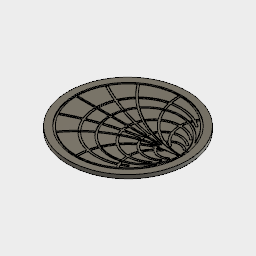
SMITH_FINAL_MODEL v0 (Autodesk Fusion 360 design; units mm, degrees)
Autodesk Fusion 360 part; units mm, degrees
note: some values were not read from the file. Chosen so that the rebuilt part matches the saved one: which face or edge a step refers to; a direction; that a step has no effect; add or cut. Set by a fixed rule: which sketch regions a step uses.
cylinder "CylinderPrimitive1" add diameter 355.6 height 12.7 placed x (1, 0, 0) y (0, 0, -1) z (0, 1, 0) at (0, 0, 0)
sketch "Smith Chart Overlay" plane through (0, 12.7, 0) normal (0, 1, 0) x (-1, 0, 0)
  circle A0 centre (0, 0) radius 177.8
  circle A1 centre (0, 0) radius 177.8
  line L0 (0, 0) -> (-177.8, 0)
  line L1 (0, 0) -> (-118.5333, 0) construction
  line L2 (0, 0) -> (-88.9, 0)
  line L3 (0, 0) -> (-59.2667, 0)
  circle A2 centre (-118.5333, 0) radius 59.2667 construction
  circle A3 centre (-88.9, 0) radius 88.9 construction
  circle A4 centre (-59.2667, 0) radius 118.5333 construction
  arc A5 (-106.68, -142.24) -> (-177.8, 0) centre (-177.8, -88.9) ccw construction
  line L4 (-177.8, 0) -> (-177.8, -88.9)
  line L5 (-177.8, 0) -> (-177.8, 88.9)
  line L6 (-177.8, 177.8) -> (-177.8, 0)
  line L7 (-177.8, 0) -> (-177.8, -177.8)
  line L8 (-177.8, 0) -> (-177.8, -355.6)
  arc A6 (-177.8, 0) -> (-106.68, 142.24) centre (-177.8, 88.9) ccw construction
  arc A7 (0, -177.8) -> (-177.8, 0) centre (-177.8, -177.8) ccw construction
  arc A8 (-177.8, 0) -> (0, 177.8) centre (-177.8, 177.8) ccw construction
  line L9 (-177.8, 355.6) -> (-177.8, 0)
  arc A9 (106.68, -142.24) -> (-177.8, 0) centre (-177.8, -355.6) ccw
  arc A10 (-177.8, 0) -> (106.68, 142.24) centre (-177.8, 355.6) ccw construction
  line L10 (-13.7583, 0) -> (-73.025, 0)
  line L11 (0, 0) -> (-59.2667, 0)
  line L12 (0, 0) -> (-35.56, 0)
  circle A11 centre (-35.56, 0) radius 142.24 construction
  line L13 (-177.8, 0) -> (-177.8, -711.2)
  arc A12 (156.8824, -83.6706) -> (-177.8, 0) centre (-177.8, -711.2) ccw construction
  arc A13 (-177.8, 0) -> (156.8824, 83.6706) centre (-177.8, 711.2) ccw construction
  line L14 (0, 0) -> (-142.24, 0) construction
  circle A14 centre (-142.24, 0) radius 35.56 construction
  line L15 (-35.56, 0) -> (177.8, 0) construction
  line L16 (-142.24, 0) -> (-165.0975, 27.2405) construction
  line L17 (-142.24, 0) -> (-152.4, 0) construction
  arc A15 (-165.0975, -27.2405) -> (-165.0975, 27.2405) centre (-142.24, 0) ccw
  line L18 (-142.24, 0) -> (-165.0975, -27.2405) construction
  line L19 (-142.24, 0) -> (-165.0975, 27.2405) construction
  line L20 (-118.5333, 0) -> (-156.6292, 45.4009) construction
  line L21 (-118.5333, 0) -> (-149.1382, 0) construction
  arc A16 (-156.6292, -45.4009) -> (-156.6292, 45.4009) centre (-118.5333, 0) ccw
  line L22 (-118.5333, 0) -> (-156.6292, -45.4009) construction
  line L23 (-118.5333, 0) -> (-156.6292, 45.4009) construction
  line L24 (-88.9, 0) -> (-146.0438, -68.1014) construction
  line L25 (-88.9, 0) -> (-123.6401, 0) construction
  arc A17 (-146.0438, -68.1014) -> (-146.0438, 68.1014) centre (-88.9, 0) ccw
  line L26 (-88.9, 0) -> (-146.0438, -68.1014) construction
  line L27 (-88.9, 0) -> (-146.0438, 68.1014) construction
  line L28 (-35.56, 0) -> (214.1255, 0) construction
  line L29 (-59.2667, 0) -> (59.2667, 0) construction
  arc A18 (52.8595, 38.4432) -> (-92.456, 113.792) centre (-59.2667, 0) ccw
  line L30 (-177.8, -711.2) -> (-177.8, 711.2)
  line L31 (-59.2667, 0) -> (-177.7955, 1.0344) construction
  line L32 (-59.2667, 0) -> (75.6719, 0) construction
  arc A19 (-177.7955, -1.0344) -> (-177.7955, 1.0344) centre (-59.2667, 0) ccw construction
  line L33 (-59.2667, 0) -> (-177.7955, -1.0344) construction
  line L34 (-59.2667, 0) -> (-177.7955, 1.0344) construction
  arc A20 (-92.456, 113.792) -> (-97.8899, 127.8562) centre (-177.8, 88.9) ccw
  arc A21 (-60.0841, 9.8097) -> (-62.4703, 19.2216) centre (-118.5333, 0) ccw
  arc A22 (-95.7385, -54.7077) -> (-116.4897, -24.5241) centre (-177.8, -88.9) ccw
  arc A23 (-92.456, -113.792) -> (-95.7385, -54.7077) centre (-177.8, -88.9) ccw
  circle A24 centre (106.68, 0) radius 2.54 construction
  circle A25 centre (59.2667, 0) radius 2.54 construction
  circle A26 centre (52.8595, -38.4432) radius 2.54 construction
  circle A27 centre (95.7385, -54.7077) radius 2.54 construction
  circle A28 centre (67.4414, -98.0965) radius 2.54 construction
  circle A29 centre (35.56, -71.12) radius 2.54 construction
  circle A30 centre (52.8595, 38.4432) radius 2.54 construction
  circle A31 centre (95.7385, 54.7077) radius 2.54 construction
  circle A32 centre (67.4414, 98.0965) radius 2.54 construction
  circle A33 centre (-97.8899, 127.8562) radius 2.54 construction
  circle A34 centre (-88.9, 88.9) radius 2.54 construction
  circle A35 centre (-13.6769, 109.4154) radius 2.54 construction
  circle A36 centre (-92.456, 113.792) radius 2.54 construction
  circle A37 centre (35.56, 71.12) radius 2.54 construction
  circle A38 centre (-2.7354, 21.8831) radius 2.54 construction
  circle A39 centre (-10.4588, 41.8353) radius 2.54 construction
  circle A40 centre (-35.56, 71.12) radius 2.54 construction
  circle A41 centre (0, 0) radius 7.62
  circle A42 centre (-2.7354, -21.8831) radius 2.54 construction
  circle A43 centre (-10.4588, -41.8353) radius 2.54 construction
  circle A44 centre (-35.56, -71.12) radius 2.54 construction
  circle A45 centre (-88.9, -88.9) radius 2.54 construction
  circle A46 centre (-95.7385, -54.7077) radius 2.54 construction
  circle A47 centre (-95.7385, 54.7077) radius 2.54 construction
  circle A48 centre (-116.4897, -24.5241) radius 2.54 construction
  circle A49 centre (-116.4897, 24.5241) radius 2.54 construction
  circle A50 centre (-71.12, 35.56) radius 2.54 construction
  circle A51 centre (-4.3366, 138.7707) radius 2.54 construction
  circle A52 centre (-71.12, -35.56) radius 2.54 construction
  circle A53 centre (-92.456, -113.792) radius 2.54 construction
  circle A54 centre (-13.6769, -109.4154) radius 2.54 construction
  circle A55 centre (156.8824, -83.6706) radius 2.54 construction
  circle A56 centre (106.68, -142.24) radius 2.54 construction
  circle A57 centre (0, -177.8) radius 2.54 construction
  circle A58 centre (-106.68, -142.24) radius 2.54 construction
  circle A59 centre (-106.68, 142.24) radius 2.54 construction
  circle A60 centre (0, 177.8) radius 2.54 construction
  circle A61 centre (106.68, 142.24) radius 2.54 construction
  circle A62 centre (156.8824, 83.6706) radius 2.54 construction
  circle A63 centre (177.8, 0) radius 5.08 construction
  line L35 (106.68, 0) -> (172.72, 0)
  arc A64 (154.639, -82.4793) -> (95.7385, -54.7077) centre (-177.8, -711.2) ccw
  arc A65 (105.1488, -140.2135) -> (67.4414, -98.0965) centre (-177.8, -355.6) ccw
  arc A66 (-105.1852, -140.1864) -> (-177.8, 0) centre (-177.8, -88.9) ccw
  arc A67 (95.7385, 54.7077) -> (154.639, 82.4793) centre (-177.8, 711.2) ccw
  arc A68 (67.4414, 98.0965) -> (105.1488, 140.2135) centre (-177.8, 355.6) ccw
  arc A69 (-4.3366, 138.7707) -> (-0.0181, 175.2601) centre (-177.8, 177.8) ccw
  arc A70 (-97.8899, 127.8562) -> (-105.1852, 140.1864) centre (-177.8, 88.9) ccw
  line L36 (59.2667, 0) -> (0, 0)
  arc A71 (-177.7955, -1.0344) -> (-177.7955, 1.0344) centre (-59.2667, 0) ccw
  arc A72 (-177.8, 0) -> (106.68, 142.24) centre (-177.8, 355.6) ccw
  line L37 (-177.8, 0) -> (177.8, 0)
  arc A73 (-130.1525, 13.8472) -> (-106.68, 142.24) centre (-177.8, 88.9) ccw
  arc A74 (-106.68, -142.24) -> (-130.1525, -13.8472) centre (-177.8, -88.9) ccw
  arc A75 (0, -177.8) -> (-177.8, 0) centre (-177.8, -177.8) ccw
  arc A76 (-177.8, 0) -> (0, 177.8) centre (-177.8, 177.8) ccw
  circle A77 centre (-4.3366, -138.7707) radius 2.54
  circle A78 centre (-59.2667, 0) radius 2.54 construction
  line L38 (-35.56, 0) -> (-117.1455, -116.5162) construction
  line L39 (-35.56, 0) -> (97.8671, 0) construction
  line L40 (-35.56, 0) -> (-117.1455, -116.5162) construction
  arc A79 (-117.1455, -116.5162) -> (-117.1455, 116.5162) centre (-35.56, 0) ccw
  line L41 (-35.56, 0) -> (-117.1455, -116.5162) construction
  line L42 (-35.56, 0) -> (-117.1455, 116.5162) construction
  circle A80 centre (-117.1455, 116.5162) radius 3.175
  circle A81 centre (-177.7955, 1.0344) radius 3.175
  circle A82 centre (-146.0438, 68.1014) radius 3.175
  circle A83 centre (-156.6292, 45.4009) radius 3.175
  circle A84 centre (-165.0975, 27.2405) radius 3.175
  circle A85 centre (-165.0975, -27.2405) radius 3.175
  circle A86 centre (-156.6292, -45.4009) radius 3.175
  circle A87 centre (-146.0438, -68.1014) radius 3.175
  circle A88 centre (-177.7955, -1.0344) radius 3.175
  circle A89 centre (-117.1455, -116.5162) radius 3.175
  circle A90 centre (-130.1525, 13.8472) radius 3.175
  circle A91 centre (-130.1525, -13.8472) radius 3.175
  arc A92 (156.8824, -83.6706) -> (-60.0841, -9.8097) centre (-177.8, -711.2) ccw
  arc A93 (-60.0841, 9.8097) -> (156.8824, 83.6706) centre (-177.8, 711.2) ccw
  circle A94 centre (0, 0) radius 3.175
  circle A95 centre (59.2667, 0) radius 19.812 construction
  line L43 (65.2043, -20.3795) -> (50.0176, -19.1059)
  line L44 (65.2043, 20.3795) -> (50.0176, 19.1059)
  line L45 (50.0176, -19.1059) -> (65.2043, -20.3795)
  line L46 (65.2043, -20.3795) -> (64.939, -23.5434)
  line L47 (64.939, -23.5434) -> (49.7523, -22.2698)
  line L48 (49.7523, -22.2698) -> (50.0176, -19.1059)
  line L49 (65.2043, -20.3795) -> (50.0176, -19.1059)
  line L50 (50.0176, -19.1059) -> (50.2829, -15.942)
  line L51 (50.2829, -15.942) -> (65.4696, -17.2156)
  line L52 (65.4696, -17.2156) -> (65.2043, -20.3795)
  line L53 (65.2043, 20.3795) -> (50.0176, 19.1059)
  line L54 (50.0176, 19.1059) -> (49.7523, 22.2698)
  line L55 (49.7523, 22.2698) -> (64.939, 23.5434)
  line L56 (64.939, 23.5434) -> (65.2043, 20.3795)
  line L57 (65.2043, 20.3795) -> (50.0176, 19.1059)
  line L58 (50.0176, 19.1059) -> (50.2829, 15.942)
  line L59 (50.2829, 15.942) -> (65.4696, 17.2156)
  line L60 (65.4696, 17.2156) -> (65.2043, 20.3795)
  circle A96 centre (0, 0) radius 19.812 construction
  line L61 (22.987, -7.62) -> (16.637, -7.62)
  line L62 (16.637, -7.62) -> (16.637, 7.62)
  line L63 (16.637, 7.62) -> (22.987, 7.62)
  line L64 (22.987, 7.62) -> (22.987, -7.62)
  line L65 (22.987, -7.62) -> (16.637, 7.62) construction
  line L66 (16.637, -7.62) -> (22.987, 7.62) construction
  line L67 (-16.637, -7.62) -> (-22.987, -7.62)
  line L68 (-22.987, -7.62) -> (-22.987, 7.62)
  line L69 (-22.987, 7.62) -> (-16.637, 7.62)
  line L70 (-16.637, 7.62) -> (-16.637, -7.62)
  line L71 (-16.637, -7.62) -> (-22.987, 7.62) construction
  line L72 (-22.987, -7.62) -> (-16.637, 7.62) construction
  circle A97 centre (35.56, -71.12) radius 19.812 construction
  line L73 (55.8124, -77.4778) -> (46.3323, -89.4104)
  line L74 (52.5378, -58.379) -> (39.6243, -50.2859)
  line L75 (23.7858, -53.4579) -> (14.985, -65.8999)
  line L76 (28.0824, -90.9862) -> (16.6972, -80.8553)
  circle A98 centre (35.56, 71.12) radius 19.812 construction
  line L77 (55.8124, 77.4778) -> (46.3323, 89.4104)
  line L78 (52.5378, 58.379) -> (39.6243, 50.2859)
  line L79 (23.7858, 53.4579) -> (14.985, 65.8999)
  line L80 (28.0824, 90.9862) -> (16.6972, 80.8553)
  line L81 (52.5378, 58.379) -> (39.6243, 50.2859)
  line L82 (39.6243, 50.2859) -> (41.3103, 47.5955)
  line L83 (41.3103, 47.5955) -> (54.2239, 55.6887)
  line L84 (54.2239, 55.6887) -> (52.5378, 58.379)
  line L85 (52.5378, 58.379) -> (39.6243, 50.2859)
  line L86 (39.6243, 50.2859) -> (37.9382, 52.9762)
  line L87 (37.9382, 52.9762) -> (50.8517, 61.0693)
  line L88 (50.8517, 61.0693) -> (52.5378, 58.379)
  line L89 (23.7858, 53.4579) -> (14.985, 65.8999)
  line L90 (14.985, 65.8999) -> (12.3929, 64.0664)
  line L91 (12.3929, 64.0664) -> (21.1937, 51.6244)
  line L92 (21.1937, 51.6244) -> (23.7858, 53.4579)
  line L93 (14.985, 65.8999) -> (23.7858, 53.4579)
  line L94 (23.7858, 53.4579) -> (26.3779, 55.2914)
  line L95 (26.3779, 55.2914) -> (17.5771, 67.7334)
  line L96 (17.5771, 67.7334) -> (14.985, 65.8999)
  line L97 (16.6972, 80.8553) -> (28.0824, 90.9862)
  line L98 (28.0824, 90.9862) -> (25.9718, 93.3581)
  line L99 (25.9718, 93.3581) -> (14.5866, 83.2272)
  line L100 (14.5866, 83.2272) -> (16.6972, 80.8553)
  line L101 (28.0824, 90.9862) -> (16.6972, 80.8553)
  line L102 (16.6972, 80.8553) -> (18.8078, 78.4834)
  line L103 (18.8078, 78.4834) -> (30.193, 88.6143)
  line L104 (30.193, 88.6143) -> (28.0824, 90.9862)
  line L105 (55.8124, 77.4778) -> (46.3323, 89.4104)
  line L106 (46.3323, 89.4104) -> (43.8463, 87.4354)
  line L107 (43.8463, 87.4354) -> (53.3264, 75.5028)
  line L108 (53.3264, 75.5028) -> (55.8124, 77.4778)
  line L109 (46.3323, 89.4104) -> (55.8124, 77.4778)
  line L110 (55.8124, 77.4778) -> (58.2983, 79.4529)
  line L111 (58.2983, 79.4529) -> (48.8182, 91.3854)
  line L112 (48.8182, 91.3854) -> (46.3323, 89.4104)
  line L113 (52.5378, -58.379) -> (39.6243, -50.2859)
  line L114 (39.6243, -50.2859) -> (37.9382, -52.9762)
  line L115 (37.9382, -52.9762) -> (50.8517, -61.0693)
  line L116 (50.8517, -61.0693) -> (52.5378, -58.379)
  line L117 (52.5378, -58.379) -> (39.6243, -50.2859)
  line L118 (39.6243, -50.2859) -> (41.3103, -47.5955)
  line L119 (41.3103, -47.5955) -> (54.2239, -55.6886)
  line L120 (54.2239, -55.6886) -> (52.5378, -58.379)
  line L121 (23.7858, -53.4579) -> (14.985, -65.8999)
  line L122 (14.985, -65.8999) -> (12.3929, -64.0664)
  line L123 (12.3929, -64.0664) -> (21.1937, -51.6244)
  line L124 (21.1937, -51.6244) -> (23.7858, -53.4579)
  line L125 (28.0824, -90.9862) -> (16.6972, -80.8553)
  line L126 (16.6972, -80.8553) -> (14.5866, -83.2272)
  line L127 (14.5866, -83.2272) -> (25.9718, -93.3581)
  line L128 (25.9718, -93.3581) -> (28.0824, -90.9862)
  line L129 (55.8124, -77.4778) -> (46.3323, -89.4104)
  line L130 (46.3323, -89.4104) -> (48.8182, -91.3854)
  line L131 (48.8182, -91.3854) -> (58.2983, -79.4529)
  line L132 (58.2983, -79.4529) -> (55.8124, -77.4778)
  line L133 (55.8124, -77.4778) -> (46.3323, -89.4104)
  line L134 (46.3323, -89.4104) -> (43.8463, -87.4354)
  line L135 (43.8463, -87.4354) -> (53.3264, -75.5028)
  line L136 (53.3264, -75.5028) -> (55.8124, -77.4778)
  line L137 (16.6972, -80.8553) -> (28.0824, -90.9862)
  line L138 (28.0824, -90.9862) -> (30.193, -88.6143)
  line L139 (30.193, -88.6143) -> (18.8078, -78.4834)
  line L140 (18.8078, -78.4834) -> (16.6972, -80.8553)
  line L141 (23.7858, -53.4579) -> (14.985, -65.8999)
  line L142 (14.985, -65.8999) -> (17.5771, -67.7334)
  line L143 (17.5771, -67.7334) -> (26.3779, -55.2914)
  line L144 (26.3779, -55.2914) -> (23.7858, -53.4579)
  circle A99 centre (14.985, -65.8999) radius 3.175
  circle A100 centre (39.6243, -50.2859) radius 3.175
  circle A101 centre (52.5378, -58.379) radius 3.175
  circle A102 centre (23.7858, -53.4579) radius 3.175
  circle A103 centre (16.6972, -80.8553) radius 3.175
  circle A104 centre (28.0824, -90.9862) radius 3.175
  circle A105 centre (46.3323, -89.4104) radius 3.175
  circle A106 centre (55.8124, -77.4778) radius 3.175
  circle A107 centre (50.0176, 19.1059) radius 3.175
  circle A108 centre (65.2043, 20.3795) radius 3.175
  circle A109 centre (50.0176, -19.1059) radius 3.175
  circle A110 centre (65.2043, -20.3795) radius 3.175
  circle A111 centre (19.812, 7.62) radius 3.175
  circle A112 centre (19.812, -7.62) radius 3.175
  circle A113 centre (-19.812, -7.62) radius 3.175
  circle A114 centre (-19.812, 7.62) radius 3.175
  point P0 (-13.6769, 109.4154)
  point P1 (95.7385, 54.7077)
  point P2 (67.4414, 98.0965)
  point P3 (-97.8899, 127.8562)
  point P4 (106.68, 0)
  point P5 (95.7385, -54.7077)
  point P6 (67.4414, -98.0965)
  point P7 (-92.456, 113.792)
  point P8 (35.56, 71.12)
  point P9 (52.8595, 38.4432)
  point P10 (52.8595, -38.4432)
  point P11 (35.56, -71.12)
  point P12 (-13.6769, -109.4154)
  point P13 (-92.456, -113.792)
  point P14 (-35.56, 71.12)
  point P15 (-88.9, 88.9)
  point P16 (-10.4588, 41.8353)
  point P17 (-2.7354, -21.8831)
  point P18 (-88.9, -88.9)
  point P19 (-10.4588, -41.8353)
  point P20 (-35.56, -71.12)
  point P21 (-146.0438, -68.1014)
  point P22 (-2.7354, 21.8831)
  point P23 (-95.7385, 54.7077)
  point P24 (-71.12, 35.56)
  point P25 (-62.4703, 19.2216)
  point P26 (-60.0841, -9.8097)
  point P27 (-62.4703, -19.2216)
  point P28 (-71.12, -35.56)
  point P29 (-95.7385, -54.7077)
  point P30 (-60.0841, 9.8097)
  point P31 (-116.4897, 24.5241)
  point P32 (-177.8, 0)
  point P33 (-177.8, 0)
  point P34 (-177.8, 0)
  point P35 (-177.8, 0)
  point P36 (-177.8, 0)
  point P37 (-177.8, 0)
  point P38 (106.68, 142.24)
  point P39 (0, 177.8)
  point P40 (156.8824, 83.6706)
  point P41 (156.8824, -83.6706)
  point P42 (177.8, 0)
  point P43 (106.68, -142.24)
  point P44 (0, -177.8)
  point P45 (59.2667, 0)
  point P46 (-177.8, 0)
  point P47 (50.4553, 37.6238)
  point P48 (53.6575, 36.0319)
  point P49 (55.2607, 39.2713)
  point P50 (52.01, 40.837)
  point P51 (96.6944, 52.3544)
  point P52 (98.0813, 55.6888)
  point P53 (93.3921, 53.735)
  point P54 (94.7406, 57.0435)
  point P55 (104.14, 0)
  point P56 (106.6573, -2.5399)
  point P57 (106.6573, 2.5399)
  point P58 (59.2395, -2.5399)
  point P59 (56.7267, 0)
  point P60 (61.8067, 0)
  point P61 (93.3921, -53.735)
  point P62 (94.7406, -57.0435)
  point P63 (98.0813, -55.6888)
  point P64 (37.0621, -69.0718)
  point P65 (34.0143, -73.1356)
  point P66 (37.5865, -72.6512)
  point P67 (33.5226, -69.6033)
  point P68 (69.1766, -96.2417)
  point P69 (65.6733, -99.9201)
  point P70 (69.2744, -99.8548)
  point P71 (65.5958, -96.3514)
  point P72 (65.5958, 96.3514)
  point P73 (65.6733, 99.9201)
  point P74 (69.1766, 96.2417)
  point P75 (69.2744, 99.8548)
  point P76 (-12.7168, 111.7669)
  point P77 (-14.6706, 107.0778)
  point P78 (-16.0319, 110.3671)
  point P79 (-16.0319, 110.3671)
  point P80 (-90.0101, 114.477)
  point P81 (-91.7797, 111.3437)
  point P82 (-93.202, 116.22)
  point P83 (-94.8866, 113.0547)
  point P84 (-37.0985, 69.0989)
  point P85 (-34.0505, 73.1628)
  point P86 (-33.55, 69.5671)
  point P87 (-37.6136, 72.6148)
  point P88 (-86.3603, 88.8637)
  point P89 (-88.9363, 86.3603)
  point P90 (-88.9363, 91.4397)
  point P91 (-91.4397, 88.8637)
  point P92 (-12.7043, 40.648)
  point P93 (-9.2957, 39.5773)
  point P94 (-8.2219, 43.0386)
  point P95 (-11.686, 44.0592)
  point P96 (109.22, 0)
  point P97 (96.6944, -52.3544)
  point P98 (59.2395, -2.5399)
  point P99 (55.2607, -39.2713)
  point P100 (52.01, -40.837)
  point P101 (50.4553, -37.6238)
  point P102 (53.6575, -36.0319)
  point P103 (-34.0505, -73.1628)
  point P104 (-37.6136, -72.6148)
  point P105 (-33.55, -69.5671)
  point P106 (-37.0985, -69.0989)
  point P107 (-88.9363, -86.3603)
  point P108 (-88.9363, -91.4397)
  point P109 (-86.3603, -88.8637)
  point P110 (-91.4397, -88.8637)
  point P111 (-94.7951, -57.066)
  point P112 (-96.7488, -52.3773)
  point P113 (-93.4153, -53.6807)
  point P114 (-114.6756, -26.302)
  point P115 (-118.3538, -22.7989)
  point P116 (-114.8047, -22.6234)
  point P117 (-93.4153, -53.6807)
  point P118 (-118.3059, 26.2997)
  point P119 (-114.6756, 26.302)
  point P120 (-118.3059, 26.2997)
  point P121 (-118.3538, 22.7989)
  point P122 (-96.7488, 52.3773)
  point P123 (-98.1035, 55.6341)
  point P124 (-93.4153, 53.6807)
  point P125 (-94.7951, 57.066)
  point P126 (-4.3366, 138.7707)
  point P127 (-69.6399, 33.4958)
  point P128 (-73.1628, 34.0505)
  point P129 (-72.6872, 37.5589)
  point P130 (-69.0989, 37.0985)
  point P131 (-100.163, 126.7228)
  point P132 (-96.8096, 125.5574)
  point P133 (-99.0354, 130.1232)
  point P134 (-95.5969, 128.9488)
  point P135 (-12.7043, -40.648)
  point P136 (-11.686, -44.0592)
  point P137 (-8.2219, -43.0386)
  point P138 (-9.2957, -39.5773)
  point P139 (-3.3957, -24.3357)
  point P140 (-0.2747, -22.5127)
  point P141 (-2.1454, -19.4126)
  point P142 (-5.1983, -21.2622)
  point P143 (-7.62, 0)
  point P144 (-0.3266, -7.613)
  point P145 (7.62, 0)
  point P146 (-0.3266, 7.613)
  point P147 (-2.1454, 19.4126)
  point P148 (-0.2747, 22.5127)
  point P149 (-5.1983, 21.2622)
  point P150 (-3.3957, 24.3357)
  point P151 (-1.8636, 138.1911)
  point P152 (-4.9118, 136.2967)
  point P153 (-6.8195, 139.3061)
  point P154 (-3.7967, 141.2527)
  point P155 (-69.0989, -37.0985)
  point P156 (-72.6872, -37.5589)
  point P157 (-73.1628, -34.0505)
  point P158 (-1.8636, -138.1911)
  point P159 (-3.7967, -141.2527)
  point P160 (-4.9118, -136.2967)
  point P161 (-16.0319, -110.3671)
  point P162 (-12.7168, -111.7669)
  point P163 (-16.0319, -110.3671)
  point P164 (-14.6706, -107.0778)
  point P165 (-192.3786, -267.9595)
  point P166 (-210, -290)
  point P167 (-225, -285)
  point P168 (-220, -260)
  point P169 (-180, -255)
  point P170 (-215, -245)
  point P171 (-185, -235)
  point P172 (-200, -225)
  point P173 (172.72, 0)
  point P174 (154.639, 82.4793)
  point P175 (154.639, -82.4793)
  point P176 (105.1488, -140.2135)
  point P177 (-0.0181, -175.2601)
  point P178 (-105.1852, -140.1864)
  point P179 (-105.1852, 140.1864)
  point P180 (-0.0181, 175.2601)
  point P181 (105.1488, 140.2135)
  point P182 (-130.1525, -13.8472)
  point P183 (-130.1525, 13.8472)
  point P184 (-177.8, 0)
  point P185 (-4.3366, -138.7707)
  point P186 (-6.8195, -139.3061)
  point P187 (-59.3211, -2.5394)
  point P188 (-56.7267, 0)
  point P189 (-61.8067, 0)
  point P190 (-59.3211, 2.5394)
  point P191 (-117.1455, -116.5162)
  point P192 (57.6109, -19.7427)
  point P193 (57.6109, 19.7427)
  point P194 (19.812, 0)
  point P195 (-19.812, 0)
  point P196 (19.812, 0)
  point P197 (-19.812, 0)
  point P198 (51.0723, -83.4441)
  point P199 (22.3898, -85.9207)
  point P200 (46.081, -54.3324)
  point P201 (19.3854, -59.6789)
  point P202 (46.081, 54.3324)
  point P203 (51.0723, 83.4441)
  point P204 (22.3898, 85.9207)
  point P205 (19.3854, 59.6789)
  dimension "d6" = 355.6
  dimension "d7" = 177.8
  dimension "d8" = 118.5333
  dimension "d11" = 59.2667
  dimension "d12" = 118.5333
  dimension "d13" = 177.8
  dimension "d14" = 237.0667
  dimension "d15" = 88.9
  dimension "d17" = 88.9
  dimension "d18" = 88.9
  dimension "d19" = 177.8
  dimension "d20" = 177.8
  dimension "d21" = 355.6
  dimension "d22" = 88.9
  dimension "d23" = 177.8
  dimension "d24" = 355.6
  dimension "d25" = 59.2667
  dimension "d26" = 59.2667
  dimension "d31" = 35.56
  dimension "d32" = 284.48
  dimension "d33" = 711.2
  dimension "d34" = 711.2
  dimension "d35" = 142.24
  dimension "d36" = 71.12
  dimension "d54" = 130
  dimension "d55" = 100
  dimension "d56" = 130
  dimension "d57" = 100
  dimension "d58" = 130
  dimension "d59" = 100
  dimension "d64" = 118.5333
  dimension "d65" = 1422.4
  dimension "d68" = 179.5
  dimension "d69" = 1
  dimension "d79" = 5.08
  dimension "d80" = 5.08
  dimension "d81" = 5.08
  dimension "d82" = 5.08
  dimension "d83" = 5.08
  dimension "d84" = 5.08
  dimension "d85" = 5.08
  dimension "d86" = 5.08
  dimension "d87" = 5.08
  dimension "d88" = 5.08
  dimension "d89" = 5.08
  dimension "d90" = 5.08
  dimension "d91" = 5.08
  dimension "d92" = 5.08
  dimension "d93" = 5.08
  dimension "d94" = 5.08
  dimension "d95" = 5.08
  dimension "d96" = 15.24
  dimension "d97" = 5.08
  dimension "d98" = 5.08
  dimension "d99" = 5.08
  dimension "d100" = 5.08
  dimension "d101" = 5.08
  dimension "d102" = 5.08
  dimension "d104" = 5.08
  dimension "d105" = 5.08
  dimension "d106" = 5.08
  dimension "d107" = 5.08
  dimension "d108" = 5.08
  dimension "d109" = 5.08
  dimension "d110" = 5.08
  dimension "d113" = 5.08
  dimension "d114" = 5.08
  dimension "d115" = 5.08
  dimension "d116" = 5.08
  dimension "d117" = 5.08
  dimension "d118" = 5.08
  dimension "d119" = 5.08
  dimension "d120" = 5.08
  dimension "d121" = 10.16
  dimension "d284" = 5.08
  dimension "d287" = 5.08
  dimension "d288" = 125
  dimension "d290" = 110
  dimension "d299" = 6.35
  dimension "d300" = 6.35
  dimension "d301" = 6.35
  dimension "d302" = 6.35
  dimension "d303" = 6.35
  dimension "d304" = 6.35
  dimension "d305" = 6.35
  dimension "d306" = 6.35
  dimension "d307" = 6.35
  dimension "d308" = 6.35
  dimension "d309" = 6.35
  dimension "d310" = 6.35
  dimension "d333" = 6.35
  dimension "d336" = 39.624
  dimension "d351" = 15.24
  dimension "d352" = 15.24
  dimension "d353" = 3.175
  dimension "d354" = 3.175
  dimension "d355" = 3.175
  dimension "d356" = 3.175
  dimension "d357" = 39.624
  dimension "d358" = 6.35
  dimension "d359" = 15.24
  dimension "d360" = 6.35
  dimension "d361" = 15.24
  dimension "d362" = 39.624
  dimension "d363" = 15.24
  dimension "d364" = 15.24
  dimension "d365" = 15.24
  dimension "d366" = 15.24
  dimension "d367" = 39.624
  dimension "d368" = 15.24
  dimension "d369" = 15.24
  dimension "d370" = 15.24
  dimension "d371" = 15.24
  dimension "d372" = 3.175
  dimension "d373" = 3.175
  dimension "d374" = 3.175
  dimension "d375" = 3.175
  dimension "d376" = 3.175
  dimension "d377" = 3.175
  dimension "d378" = 3.175
  dimension "d379" = 3.175
  dimension "d380" = 3.175
  dimension "d381" = 3.175
  dimension "d382" = 3.175
  dimension "d383" = 3.175
  dimension "d384" = 3.175
  dimension "d385" = 3.175
  dimension "d386" = 3.175
  dimension "d387" = 3.175
  dimension "d388" = 6.35
  dimension "d389" = 6.35
  dimension "d390" = 6.35
  dimension "d391" = 6.35
  dimension "d392" = 6.35
  dimension "d393" = 6.35
  dimension "d394" = 6.35
  dimension "d395" = 6.35
  dimension "d396" = 6.35
  dimension "d397" = 6.35
  dimension "d398" = 6.35
  dimension "d399" = 6.35
  dimension "d400" = 6.35
  dimension "d401" = 6.35
  dimension "d402" = 6.35
  dimension "d403" = 6.35
  measures "d6" diameter of A1
  measures "d7" distance of A0.centre P184
  measures "d8" distance of A0.centre L1.end
  measures "d11" distance of A0.centre L3.end
  measures "d12" diameter of A2
  measures "d13" diameter of A3
  measures "d14" diameter of A4
  measures "d15" radius of A5
  measures "d17" distance of P184 A5.centre
  measures "d18" distance of P184 L5.end
  measures "d19" distance of L6.start P184
  measures "d20" distance of P184 L7.end
  measures "d21" distance of P184 L8.end
  measures "d22" radius of A6
  measures "d23" radius of A7
  measures "d24" distance of L9.start P184
  measures "d25" distance of L10.end L10.start
  measures "d26" distance of L3.end A0.centre
  measures "d31" distance of A0.centre L12.end
  measures "d32" diameter of A11
  measures "d33" distance of P184 L13.end
  measures "d34" distance of P184 A13.centre
  measures "d35" distance of A0.centre L14.end
  measures "d36" diameter of A14
  measures "d54" angle of L16 L17
  measures "d55" angle of L18 L19
  measures "d56" angle of L20 L21
  measures "d57" angle of L22 L23
  measures "d58" angle of L24 L25
  measures "d59" angle of L26 L27
  measures "d64" radius of A18
  measures "d65" distance of L13.end A13.centre
  measures "d68" angle of L31 L32
  measures "d69" angle of L33 L34
  measures "d79" diameter of A24
  measures "d80" diameter of A25
  measures "d81" diameter of A26
  measures "d82" diameter of A27
  measures "d83" diameter of A28
  measures "d84" diameter of A29
  measures "d85" diameter of A30
  measures "d86" diameter of A31
  measures "d87" diameter of A32
  measures "d88" diameter of A33
  measures "d89" diameter of A34
  measures "d90" diameter of A35
  measures "d91" diameter of A36
  measures "d92" diameter of A37
  measures "d93" diameter of A38
  measures "d94" diameter of A39
  measures "d95" diameter of A40
  measures "d96" diameter of A41
  measures "d97" diameter of A42
  measures "d98" diameter of A43
  measures "d99" diameter of A44
  measures "d100" diameter of A45
  measures "d101" diameter of A46
  measures "d102" diameter of A47
  measures "d104" diameter of A48
  measures "d105" diameter of A49
  measures "d106" diameter of A50
  measures "d107" diameter of A51
  measures "d108" diameter of A52
  measures "d109" diameter of A53
  measures "d110" diameter of A54
  measures "d113" diameter of A55
  measures "d114" diameter of A56
  measures "d115" diameter of A57
  measures "d116" diameter of A58
  measures "d117" diameter of A59
  measures "d118" diameter of A60
  measures "d119" diameter of A61
  measures "d120" diameter of A62
  measures "d121" diameter of A63
  measures "d284" diameter of A77
  measures "d287" diameter of A78
  measures "d288" angle of L38 L39
  measures "d290" angle of L41 L42
  measures "d299" diameter of A80
  measures "d300" diameter of A81
  measures "d301" diameter of A82
  measures "d302" diameter of A83
  measures "d303" diameter of A84
  measures "d304" diameter of A85
  measures "d305" diameter of A86
  measures "d306" diameter of A87
  measures "d307" diameter of A88
  measures "d308" diameter of A89
  measures "d309" diameter of A90
  measures "d310" diameter of A91
  measures "d333" diameter of A94
  measures "d336" diameter of A95
  measures "d351" distance of L43.start L43.end
  measures "d352" distance of L44.start L44.end
  measures "d353" distance of L43.end L47.end
  measures "d354" distance of L43.start L51.end
  measures "d355" distance of L44.start L55.end
  measures "d356" distance of L44.start L59.end
  measures "d357" diameter of A96
  measures "d358" distance of L62.end L63.end
  measures "d359" distance of L61.end L62.end
  measures "d360" distance of L68.end L69.end
  measures "d361" distance of L67.end L68.end
  measures "d362" diameter of A97
  measures "d363" distance of L73.start L73.end
  measures "d364" distance of L74.start L74.end
  measures "d365" distance of L75.start L75.end
  measures "d366" distance of L76.start L76.end
  measures "d367" diameter of A98
  measures "d368" distance of L77.start L77.end
  measures "d369" distance of L78.start L78.end
  measures "d370" distance of L79.start L79.end
  measures "d371" distance of L80.start L80.end
  measures "d372" distance of L78.start L83.end
  measures "d373" distance of L78.start L87.end
  measures "d374" distance of L79.start L91.end
  measures "d375" distance of L79.end L95.end
  measures "d376" distance of L80.end L99.end
  measures "d377" distance of L80.start L103.end
  measures "d378" distance of L77.start L107.end
  measures "d379" distance of L77.end L111.end
  measures "d380" distance of L74.start L115.end
  measures "d381" distance of L74.start L119.end
  measures "d382" distance of L75.start L123.end
  measures "d383" distance of L76.start L127.end
  measures "d384" distance of L73.start L131.end
  measures "d385" distance of L73.start L135.end
  measures "d386" distance of L76.end L139.end
  measures "d387" distance of L75.start L143.end
  measures "d388" diameter of A99
  measures "d389" diameter of A100
  measures "d390" diameter of A101
  measures "d391" diameter of A102
  measures "d392" diameter of A103
  measures "d393" diameter of A104
  measures "d394" diameter of A105
  measures "d395" diameter of A106
  measures "d396" diameter of A107
  measures "d397" diameter of A108
  measures "d398" diameter of A109
  measures "d399" diameter of A110
  measures "d400" diameter of A111
  measures "d401" diameter of A112
  measures "d402" diameter of A113
  measures "d403" diameter of A114
sketch "Outer Circle" plane through (0, 0, 0) normal (0, 1, 0) x (1, 0, 0)
  circle A0 centre (0, 0) radius 203.2
  circle A1 centre (0, 0) radius 177.8
  dimension "d192" = 406.4
  dimension "d193" = 355.6
  measures "d192" diameter of A0
  measures "d193" diameter of A1
extrude "Extrude1" add sketch "Outer Circle" along normal blind 12.7
pipe "Pipe18" cut square section size 6.35 path "Smith Chart Overlay" along A1
pipe "Pipe19" cut square section size 6.35 path "Smith Chart Overlay" along A71
extrude "Extrude2" add 1 faces at (168.3288, 9.525, -46.3477) along direction (0, 1, 0) blind 6.985
extrude "Extrude3" cut 1 faces at (158.1547, 13.97, 74.0336) along direction (0, 1, 0) blind 6.985
pipe "Pipe20" cut square section size 6.35 path "Smith Chart Overlay" along A17
extrude "Extrude4" add 1 faces at (139.6945, 9.525, 73.9832) along direction (0, 1, 0) blind 4.445
pipe "Pipe22" cut square section size 6.35 path "Smith Chart Overlay" along A15
pipe "Pipe23" cut square section size 6.35 path "Smith Chart Overlay" along A16
extrude "Extrude6" add 2 faces at (162.966, 9.525, 30.0797) (152.6231, 9.525, 49.5924) along direction (0, 1, 0) blind 4.445
pipe "Pipe24" cut square section size 6.35 path "Smith Chart Overlay" along A9
pipe "Pipe25" cut square section size 6.35 path "Smith Chart Overlay" along A72
extrude "Extrude7" add 1 faces at (146.7669, 9.525, -1.0583) along direction (0, 1, 0) blind 6.985
pipe "Pipe26" cut square section size 6.35 path "Smith Chart Overlay" along L37
extrude "Extrude8" add 1 faces at (59.2667, 9.525, -1.0583) along direction (0, 1, 0) blind 6.985
pipe "Pipe27" cut square section size 6.35 path "Smith Chart Overlay" along A23 A22
pipe "Pipe28" cut square section size 6.35 path "Smith Chart Overlay" along A74
pipe "Pipe29" cut square section size 6.35 path "Smith Chart Overlay" along A73
extrude "Extrude9" add 2 faces at (92.2601, 9.525, 61.7957) (106.6002, 9.525, -34.2895) along direction (0, 1, 0) blind 4.445
pipe "Pipe30" cut square section size 6.35 path "Smith Chart Overlay" along A76
pipe "Pipe31" cut square section size 6.35 path "Smith Chart Overlay" along A75
extrude "Extrude10" add 1 faces at (161.2322, 9.525, 1.0583) along direction (0, 1, 0) blind 4.445
extrude "Extrude11" [no effect]
extrude "Extrude14" cut 1 faces at (150.1548, 16.51, 1.0632) along direction (0, -1, 0) blind 7.62
pipe "Pipe32" cut square section size 6.35 path "Smith Chart Overlay" along A79
extrude "Extrude17" add 4 faces at (-45.2244, 9.525, 117.9791) (-45.2244, 9.525, -117.9791) (-107.0538, 9.525, 10.0937) (-107.0538, 9.525, -10.0937) along direction (0, 1, 0) blind 4.445
extrude "Extrude18" cut 10 faces at (115.5964, 13.97, 10.9436) (58.4332, 13.97, -4.7556) (-0.5524, 13.97, -7.4562) (58.4332, 13.97, 4.7556) (-0.5524, 13.97, 7.4562) (-5.2399, 13.97, 137.0592) (115.5964, 13.97, -10.9436) (-5.2399, 13.97, -137.0592) (-107.0538, 13.97, 10.0937) (-107.0538, 13.97, -10.0937) along direction (0, -1, 0) blind 2.54
extrude "Extrude19" cut sketch "Smith Chart Overlay" against normal blind 1.27 contours A66 A74 A91 | A66 A74 A91 | A80 | A82 | A83 | A84 | A85 | A86 | A87 | A89 | A90
extrude "Extrude20" cut sketch "Smith Chart Overlay" against normal blind 3.81 contours A0 A1 L5 L6 L9 L30 A71 A81 A88 | A0 A1 L5 L6 L9 L30 A71 A81 A88 | A0 A1 L4 L7 L8 L13 L30 A71 A81 A88 | A0 A1 L4 L7 L8 L13 L30 A71 A81 A88 | A0 A1 L0 L5 L6 L9 A9 L30 A66 A71 A72 L37 A75 A76 A88 | A0 A1 L4 L5 L6 L7 L8 L9 L13 L30 A71 A81 A88 | A0 A1 L0 L4 L7 L8 A9 L13 L30 A66 A71 A72 L37 A75 A76 A81
pipe "Pipe33" cut square section size 6.35 path "Smith Chart Overlay" along A93
pipe "Pipe34" cut square section size 6.35 path "Smith Chart Overlay" along A92
extrude "Extrude21" add 4 faces at (-1.6965, 9.525, 22.1615) (-1.6965, 9.525, -22.1615) (-111.5102, 9.525, 60.5646) (-111.5102, 9.525, -60.5646) along direction (0, 1, 0) blind 4.445
extrude "Extrude22" cut 4 faces at (-1.6965, 13.97, 22.1615) (-1.6965, 13.97, -22.1615) (-111.5102, 13.97, 60.5646) (-111.5102, 13.97, -60.5646) along direction (0, -1, 0) blind 2.54
extrude "Extrude23" cut 2 faces at (105.8083, 13.97, -3.6603) (105.8083, 13.97, 3.6603) along direction (0, -1, 0) blind 1.27
extrude "Extrude24" cut sketch "Smith Chart Overlay" against normal blind 3.81 contours A17 A41 L36 L37 A94 | L0 L2 L3 L11 L12 A17 A41 L37 A94 | L0 L2 L3 L11 L12 A17 A41 L37 A94 | A17 A41 L36 L37 A94 | A17 L36 L37 A94 | L0 L2 L3 L11 L12 A17 L37 A94 | L0 L2 L3 L11 L12 A17 L37 A94 | A17 L36 L37 A94
extrude "Extrude25" cut sketch "Smith Chart Overlay" against normal blind 6.35 contours A17 L36 L37 A94 | L0 L2 L3 L11 L12 A17 L37 A94 | L0 L2 L3 L11 L12 A17 L37 A94 | A17 L36 L37 A94
extrude "Extrude16" cut 2 faces at (138.0148, 11.8533, 70.2603) (94.0683, 11.8533, 70.5211) along direction (0, 1, 0) blind 1.27
equation "inner_body_diameter = body_diameter - 2 in"
equation "body_height = 0.5 in"
equation "d3 = body_height"
equation "d4 = inner_body_diameter"
equation "d6 = inner_body_diameter"
equation "d7 = radius"
equation "d8 = ( 2 * radius / ( radius + 2 * radius ) ) * radius"
equation "radius = inner_body_diameter / 2"
equation "d10 = ( radius / ( radius + radius ) ) * radius"
equation "d11 = ( 0.5 * radius / ( radius + 0.5 * radius ) ) * radius"
equation "d12 = 2 * ( radius / ( radius + 2 * radius ) ) * radius"
equation "d13 = 2 * ( radius / ( radius + 1 * radius ) ) * radius"
equation "d14 = 2 * ( radius / ( radius + 0.5 * radius ) ) * radius"
equation "d15 = radius / ( 2 * radius ) * radius"
equation "d17 = radius / ( 2 * radius ) * radius"
equation "d18 = radius / ( 2 * radius ) * radius"
equation "d19 = radius / ( 1 * radius ) * radius"
equation "d20 = radius / ( 1 * radius ) * radius"
equation "d21 = radius / ( 0.5 * radius ) * radius"
equation "d22 = radius / ( 2 * radius ) * radius"
equation "d23 = radius / ( 1 * radius ) * radius"
equation "d24 = radius / ( 0.5 * radius ) * radius"
equation "d25 = ( 0.5 * radius / ( radius + 0.5 * radius ) ) * radius"
equation "d26 = ( 0.5 * radius / ( radius + 0.5 * radius ) ) * radius"
equation "d31 = ( 0.25 * radius / ( radius + 0.25 * radius ) ) * radius"
equation "d32 = 2 * ( radius / ( radius + 0.25 * radius ) ) * radius"
equation "d33 = radius / ( 0.25 * radius ) * radius"
equation "d34 = radius / ( 0.25 * radius ) * radius"
equation "d35 = ( 4 * radius / ( radius + 4 * radius ) ) * radius"
equation "d36 = 2 * ( radius / ( radius + 4 * radius ) ) * radius"
equation "arc_angle1 = 260 deg"
equation "arc_angle5 = 250 deg"
equation "arc_angle2 = 260 deg"
equation "arc_angle3 = 260 deg"
equation "arc_angle4 = 359 deg"
equation "d54 = arc_angle1 / 2"
equation "d55 = 360 deg - arc_angle1"
equation "d56 = arc_angle2 / 2"
equation "d57 = 360 deg - arc_angle2"
equation "d58 = arc_angle3 / 2"
equation "d59 = 360 deg - arc_angle3"
equation "d64 = ( radius / ( radius + 0.5 * radius ) ) * radius"
equation "d65 = 2 * radius / ( 0.25 * radius ) * radius"
equation "d68 = arc_angle4 / 2"
equation "d69 = 360 deg - arc_angle4"
equation "distance_guide = 0.1 in"
equation "distance_circle = 2 * distance_guide"
equation "d79 = distance_circle"
equation "d80 = distance_circle"
equation "d81 = distance_circle"
equation "d82 = distance_circle"
equation "d83 = distance_circle"
equation "d84 = distance_circle"
equation "d85 = distance_circle"
equation "d86 = distance_circle"
equation "d87 = distance_circle"
equation "d88 = distance_circle"
equation "d89 = distance_circle"
equation "d90 = distance_circle"
equation "d91 = distance_circle"
equation "d92 = distance_circle"
equation "d93 = distance_circle"
equation "d94 = distance_circle"
equation "d95 = distance_circle"
equation "d96 = 3 * distance_circle"
equation "d97 = distance_circle"
equation "d98 = distance_circle"
equation "d99 = distance_circle"
equation "d100 = distance_circle"
equation "d101 = distance_circle"
equation "d102 = distance_circle"
equation "d104 = distance_circle"
equation "d105 = distance_circle"
equation "d106 = distance_circle"
equation "d107 = distance_circle"
equation "d108 = distance_circle"
equation "d109 = distance_circle"
equation "d110 = distance_circle"
equation "d113 = distance_circle"
equation "d114 = distance_circle"
equation "d115 = distance_circle"
equation "d116 = distance_circle"
equation "d117 = distance_circle"
equation "d118 = distance_circle"
equation "d119 = distance_circle"
equation "d120 = distance_circle"
equation "d121 = 2 * distance_circle"
equation "trough_width = 0.25 in"
equation "body_diameter = 16 in"
equation "d192 = body_diameter"
equation "d193 = inner_body_diameter"
equation "d194 = body_height"
equation "d198 = trough_width"
equation "d202 = trough_width"
equation "trough_depth1 = 0.15 in"
equation "trough_depth2 = 0.05 in"
equation "d206 = trough_width / 2 + trough_depth1"
equation "d208 = trough_width / 2 + trough_depth1"
equation "d212 = trough_width"
equation "d214 = trough_width / 2 + trough_depth2"
equation "d224 = trough_width"
equation "d228 = trough_width"
equation "d230 = trough_width / 2 + trough_depth2"
equation "d234 = trough_width"
equation "d238 = trough_width"
equation "d240 = trough_width / 2 + trough_depth1"
equation "d244 = trough_width"
equation "d246 = trough_width / 2 + trough_depth1"
equation "d250 = trough_width"
equation "d254 = trough_width"
equation "d258 = trough_width"
equation "d260 = trough_width / 2 + trough_depth2"
equation "d264 = trough_width"
equation "d268 = trough_width"
equation "d270 = trough_width / 2 + trough_depth2"
equation "d272 = trough_width / 2 + trough_depth2"
equation "d278 = -2 * trough_depth1"
equation "d282 = -trough_depth2"
equation "d284 = distance_circle"
equation "d287 = distance_circle"
equation "d288 = arc_angle5 / 2"
equation "d290 = 360 deg - arc_angle5"
equation "d293 = trough_width"
equation "d295 = trough_width / 2 + trough_depth2"
equation "d297 = -2 * trough_depth2"
equation "d299 = trough_width"
equation "d300 = trough_width"
equation "d301 = trough_width"
equation "d302 = trough_width"
equation "d303 = trough_width"
equation "d304 = trough_width"
equation "d305 = trough_width"
equation "d306 = trough_width"
equation "d307 = trough_width"
equation "d308 = trough_width"
equation "d309 = trough_width"
equation "d310 = trough_width"
equation "d311 = -trough_depth2"
equation "d313 = -trough_depth1"
equation "d317 = trough_width"
equation "d321 = trough_width"
equation "d323 = trough_width / 2 + trough_depth2"
equation "d325 = -2 * trough_depth2"
equation "d327 = -trough_depth2"
equation "end_circle_depth = 0.1 in"
equation "d331 = -trough_depth1"
equation "d333 = trough_width"
equation "d334 = -end_circle_depth - trough_depth1"
equation "d336 = 3 * distance_circle + 2 * 0.03 * body_diameter"
equation "d351 = 3 * distance_circle"
equation "d352 = 3 * distance_circle"
equation "d353 = trough_width / 2"
equation "d354 = trough_width / 2"
equation "d355 = trough_width / 2"
equation "d356 = trough_width / 2"
equation "d357 = 3 * distance_circle + 2 * 0.03 * body_diameter"
equation "d358 = trough_width"
equation "d359 = 3 * distance_circle"
equation "d360 = trough_width"
equation "d361 = 3 * distance_circle"
equation "d362 = 3 * distance_circle + 2 * 0.03 * body_diameter"
equation "d363 = 3 * distance_circle"
equation "d364 = 3 * distance_circle"
equation "d365 = 3 * distance_circle"
equation "d366 = 3 * distance_circle"
equation "d367 = 3 * distance_circle + 2 * 0.03 * body_diameter"
equation "d368 = 3 * distance_circle"
equation "d369 = 3 * distance_circle"
equation "d370 = 3 * distance_circle"
equation "d371 = 3 * distance_circle"
equation "d372 = trough_width / 2"
equation "d373 = trough_width / 2"
equation "d374 = trough_width / 2"
equation "d375 = trough_width / 2"
equation "d376 = trough_width / 2"
equation "d377 = trough_width / 2"
equation "d378 = trough_width / 2"
equation "d379 = trough_width / 2"
equation "d380 = trough_width / 2"
equation "d381 = trough_width / 2"
equation "d382 = trough_width / 2"
equation "d383 = trough_width / 2"
equation "d384 = trough_width / 2"
equation "d385 = trough_width / 2"
equation "d386 = trough_width / 2"
equation "d387 = trough_width / 2"
equation "d388 = trough_width"
equation "d389 = trough_width"
equation "d390 = trough_width"
equation "d391 = trough_width"
equation "d392 = trough_width"
equation "d393 = trough_width"
equation "d394 = trough_width"
equation "d395 = trough_width"
equation "d396 = trough_width"
equation "d397 = trough_width"
equation "d398 = trough_width"
equation "d399 = trough_width"
equation "d400 = trough_width"
equation "d401 = trough_width"
equation "d402 = trough_width"
equation "d403 = trough_width"
